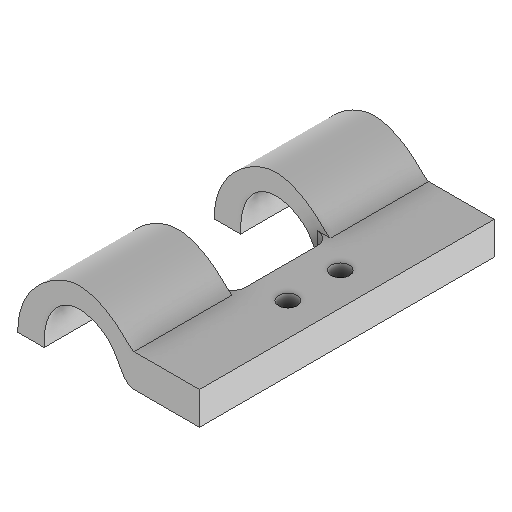
# Autodesk Inventor part: 60_Planktoscope_Sampleclamp
Saved by Autodesk Inventor 2024.1 (Build 281209000, 209)
## iProperties
Created: 2024-04-13
Part Number: 60_Planktoscope_Sampleclamp
Material: Generisch
Document SubType Name: Modeling
Designer: diederichbenedict
Density: 1 g/cm^3
Appearance: Vorgabe
Author: diederichbenedict
Autodesk Inventor part; units mm, degrees
ref_plane "YZ Plane" through (0, 0, 0) normal (1, 0, 0) x (0, 1, 0)
ref_plane "XZ Plane" through (0, 0, 0) normal (0, 1, 0) x (-1, 0, 0)
ref_plane "XY Plane" through (0, 0, 0) normal (0, 0, 1) x (1, 0, 0)
sketch "Skizze1" plane through (0, 0, 0) normal (0, 0, 1) x (1, 0, 0)
  circle A0 centre (-16.9417, 54.3) radius 1.65 projected
  circle A1 centre (-5.6501, 4) radius 1.4 projected
  circle A2 centre (-5.6501, -4) radius 1.4 projected
  circle A3 centre (-16.9417, 18.1) radius 1.65 projected
  line L0 (-0.6501, -22.5) -> (-10.6501, -22.5)
  line L1 (-10.6501, -22.5) -> (-10.6501, 22.5)
  line L2 (-10.6501, 22.5) -> (-0.6501, 22.5)
  line L3 (-0.6501, 22.5) -> (-0.6501, -22.5)
  line L4 (-0.6501, -22.5) -> (-10.6501, 22.5) construction
  line L5 (-10.6501, -22.5) -> (-0.6501, 22.5) construction
  point P0 (0, 0)
  point P1 (-5.6501, 0)
  dimension "d0" = 10
  dimension "d1" = 45
  constraints: 12 end point, 2 midpoint, 2 parallel, 1 horizontal, 1 perpendicular
  measures "d0" distance of L1.end L2.end
  measures "d1" distance of L0.end L1.end
extrude "Extrusion1" add sketch "Skizze1" along normal blind 5 contours L0 L1 L2 L3
sketch "Skizze2" plane through (-10.6501, -22.5, 0) normal (0, -1, 0) x (1, 0, 0)
  line L0 (0, 0) -> (10, 0) projected
  line L1 (10, 0) -> (10, 5) projected
  line L2 (0, 5) -> (10, 5) projected
  line L3 (0, 0) -> (0, 5) projected
  line L4 (0, 0) -> (-1.6429, 0) construction
  line L5 (-1.6429, 0) -> (-2.7402, 4.5123) construction
  line L6 (-2.7402, 4.5123) -> (-5.3021, 5.5945) construction
  line L7 (-5.3021, 5.5945) -> (-9.43, 7.7902) construction
  line L8 (-9.43, 7.7902) -> (-13.8799, 3.8379) construction
  line L9 (-13.8799, 3.8379) -> (-13.7228, -1.3116) construction
  spline S0 degree 4 poles (0, 0) (-1.6429, 0) (-2.7402, 4.5123) (-5.3021, 5.5945) (-9.43, 7.7902) (-13.8799, 3.8379) (-13.7228, -1.3116) knots 1 1 1 1 1 2 3 4 4 4 4 4
  line L10 (0, 5) -> (-0.4655, 5) construction
  line L11 (-0.4655, 5) -> (-2.7402, 8.0244) construction
  line L12 (-2.7402, 8.0244) -> (-7.1757, 9.8395) construction
  line L13 (-7.1757, 9.8395) -> (-10.7181, 10.2483) construction
  line L14 (-10.7181, 10.2483) -> (-17.7424, 4.5123) construction
  line L15 (-17.7424, 4.5123) -> (-17.7424, -1.3116) construction
  spline S1 degree 4 poles (0, 5) (-0.4655, 5) (-2.7402, 8.0244) (-7.1757, 9.8395) (-10.7181, 10.2483) (-17.7424, 4.5123) (-17.7424, -1.3116) knots 1 1 1 1 1 2 3 4 4 4 4 4
  line L16 (-17.7424, -1.3116) -> (-13.7228, -1.3116)
  point P0 (10.6501, 0)
  constraints: 3 horizontal, 2 end point, 6 other
extrude "Extrusion2" add sketch "Skizze2" against normal up to surface (45 mm away) contours S0 L16 S1 L3
sketch "Skizze3" plane through (0, 0, 5) normal (0, 0, 1) x (1, 0, 0)
  line L0 (-0.6501, 22.5) -> (-10.6501, 22.5) projected
  line L1 (-10.6501, 22.5) -> (-10.6501, -22.5) projected
  line L2 (-10.6501, -22.5) -> (-0.6501, -22.5) projected
  line L3 (-0.6501, -22.5) -> (-0.6501, 22.5) projected
  circle A0 centre (-5.6501, -4) radius 1.4 projected
  circle A1 centre (-5.6501, 4) radius 1.4 projected
  line L4 (-42.8998, -7.5) -> (-10.6501, -7.5)
  line L5 (-10.6501, -7.5) -> (-10.6501, 7.5)
  line L6 (-10.6501, 7.5) -> (-42.8998, 7.5)
  line L7 (-42.8998, 7.5) -> (-42.8998, -7.5)
  line L8 (-42.8998, -7.5) -> (-10.6501, 7.5) construction
  line L9 (-10.6501, -7.5) -> (-42.8998, 7.5) construction
  line L10 (-10.6501, 22.5) -> (-42.8998, 7.5)
  line L11 (-42.8998, -7.5) -> (-10.6501, -22.5)
  line L12 (-42.8998, 22.5) -> (-10.6501, 22.5)
  line L13 (-10.6501, 22.5) -> (-10.6501, -22.5)
  line L14 (-10.6501, -22.5) -> (-42.8998, -22.5)
  line L15 (-42.8998, -22.5) -> (-42.8998, 22.5)
  point P0 (0, 0)
  point P1 (-26.775, 0)
  point P2 (-10.6501, -7.5)
  dimension "d6" = 15
  constraints: 24 end point, 4 parallel, 2 horizontal, 2 midpoint, 2 perpendicular, 1 point on line
  measures "d6" distance of L5.end L4.end
extrude "Extrusion3" cut sketch "Skizze3" along normal through all both and the other way through all contours L1 L4 L7 L6
fillet "Rundung1" radius 2 2 edges at (-10.6501, 7.5, 2.5) (-10.6501, -7.5, 2.5)
